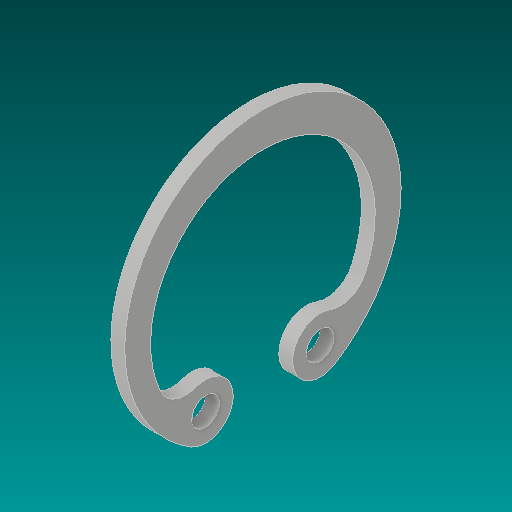
# Autodesk Inventor part: RRING-C-INT-S-19
Saved by Autodesk Inventor 2020 (Build 240168000, 168)
## iProperties
Created: 2022-11-02
Part Number: RRING-C-INT-S-19
Material: Generic
Catalog Web Link: www.cadenas.de
Description: RRING_C_INT-Retaining Rings - C  (Internal)
Vendor: MISUMI
Document SubType Name: Modeling
Designer: psAdmin
Manufacturer: MISUMI
Mass: 0.110311 g
Surface Area: 3.39751 cm^2
Volume: 0.110311 cm^3
Density: 1 g/cm^3
Appearance: PSOLRGB-175-175-175
Category: PARTsolutions
Company: MISUMI
PSOL_IDENT_0: {$CADENAS_DATA/23d-libs/misumi/metric/accessories/rring_c_int.prj},180 {VTYP=3D},{NB=RRING-C-INT-S-1
PSOL_IDENT_1: 9},{LINA=RRING-C-INT-S-19},{NN=RRING_C_INT},{DATE=30.06.2021 13:30:10},{GEOMDATE=05.03.2015 00:00:00
PSOL_IDENT_2: },{VERSION=},{LINEID=90},{WBVAR=MAT},{WBNUMERIC=}  {NB=RRING-C-INT-S-19},{LINA=RRING-C-INT-S-19},{KT=
PSOL_IDENT_3: DUMMY},{PN=RRING-C-INT-S-19},{TYPE=RRING-C-INT},{MAT=-S},{HARD=36~44HRC},{NO=19},{DD3=20.5},{DD3TOL=
PSOL_IDENT_4: +0.2/-0.2},{TT=1.00},{TTTOL=+0.05/-0.05},{BB=2.5},{AA=4.0},{DD0=2.0},{DD4=11},{DD1=19},{DD2=20.0},{D
PSOL_IDENT_5: D2TOL=+0.21/0},{MM=1.15},{MMTOL=+0.14/0},{NN=1.5},{A2=8.30}
NB: RRING-C-INT-S-19
NN: 1.5
NT: Retaining Rings - C  (Internal)
NBSYN: $PN.
LINA: RRING-C-INT-S-19
CATALOG: Misumi
PN: RRING-C-INT-S-19
MAT: 304 Stainless Steel-CSP
HARD: 36~44HRC
NO: 19
DD3: 20.5
DD3TOL: +0.2/-0.2
TT: 1
TTTOL: +0.05/-0.05
BB: 2.5
AA: 4
DD0: 2
DD4: 11
DD1: 19
DD2: 20
DD2TOL: +0.21/0
MM: 1.15
MMTOL: +0.14/0
SUPPLIER: MISUMI
ARTICLENO: RRING-C-INT-S-19
BOMINFO: RRING-C-INT-S-19
CREATOR: CADENAS GmbH
d2: 0.000 mm
Title: RRING-C-INT-S-19
Author: Cadenas PARTsolutions
Comments: Retaining Rings - C  (Internal)
Autodesk Inventor part; units mm, degrees
sketch "Sketch_3" plane through (0, 0, 0) normal (1, 0, 0) x (0, 1, 0)
  arc A0 (-8.5493, -5.1875) -> (-8.5493, 5.1875) centre (0, 0) ccw
  arc A1 (-8.5493, 5.1875) -> (-7.4165, 2.2351) centre (-6.8394, 4.15) ccw
  arc A2 (-7.4165, 2.2351) -> (-4.975, 4.874) centre (-6.8394, 4.15) ccw
  arc A3 (-3.9223, 7.4259) -> (-4.975, 4.874) centre (-3.1107, 5.5979) ccw
  arc A4 (-3.9223, -7.4259) -> (-3.9223, 7.4259) centre (-0.625, 0) ccw
  arc A5 (-4.975, -4.874) -> (-3.9223, -7.4259) centre (-3.1107, -5.5979) ccw
  arc A6 (-4.975, -4.874) -> (-7.4165, -2.2351) centre (-6.8394, -4.15) ccw
  arc A7 (-7.4165, -2.2351) -> (-8.5493, -5.1875) centre (-6.8394, -4.15) ccw
  circle A8 centre (-6.8394, -4.15) radius 1
  circle A9 centre (-6.8394, 4.15) radius 1
  constraints: 16 point on circle, 10 centre point
extrude "Extrusion1" add sketch "Sketch_3" along normal mid plane 1
ref_plane "rr_XY" through (-0.5, 0, 0) normal (1, 0, 0) x (0, 0, -1)
ref_plane "rr_YZ" through (-0.5, 0, 0) normal (0, 0, -1) x (0, 1, 0)
ref_plane "rr_ZX" through (-0.5, 0, 0) normal (0, 1, 0) x (1, 0, 0)
body "Solid1"
